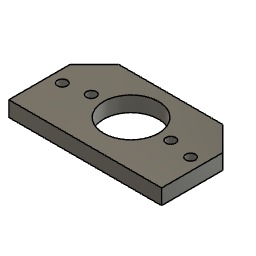
move_base_sonar_plate (Autodesk Fusion 360 design; units mm, degrees)
Autodesk Fusion 360 part; units mm, degrees
sketch "スケッチ1" plane through (0, 0, 0) normal (0, 1, 0) x (1, 0, 0)
  line L0 (-25, 0) -> (25, 0)
  line L1 (25, 0) -> (25, 28)
  line L2 (25, 28) -> (-25, 28)
  line L3 (-25, 28) -> (-25, 0)
  line L4 (-13, 15) -> (13, 15)
  circle A0 centre (0, 15) radius 9
  line L5 (-21, 13.5) -> (21, 13.5)
  point P0 (0, 15)
  point P1 (0, 13.5)
  dimension "d1" = 50
  dimension "d2" = 26
  dimension "d3" = 15
  dimension "d4" = 28
  dimension "d5" = 18
  dimension "d12" = 13.5
  dimension "d13" = 42
  constraint horizontal L0
  constraint vertical L1
  constraint horizontal L2
  constraint vertical L3
  constraint midpoint origin L0
  constraint perpendicular L3 L4
  constraint midpoint L4 P0
  constraint vertical origin A0.centre
  constraint coincident P0 A0.centre
  constraint horizontal L5
  constraint midpoint L5 P1
  constraint vertical origin P1
  measures "d1" distance of L0.start L0.end
  measures "d2" distance of L4.start L4.end
  measures "d3" distance of origin L4
  measures "d4" distance of L0 L2
  measures "d5" diameter of A0
  measures "d12" distance of L0 L5
  measures "d13" distance of L5.start L5.end
extrude "押し出し1" add sketch "スケッチ1" along normal blind 5
hole "穴1" at (-13, 0, -15) at (13, 0, -15) at (-21, 0, -13.5) at (21, 0, -13.5) direction (0, 1, 0) diameter 3.2 end through all
chamfer "面取り1" distance 8 angle 45 2 edges at (-25, 2.5, -28) (25, 2.5, -28)
